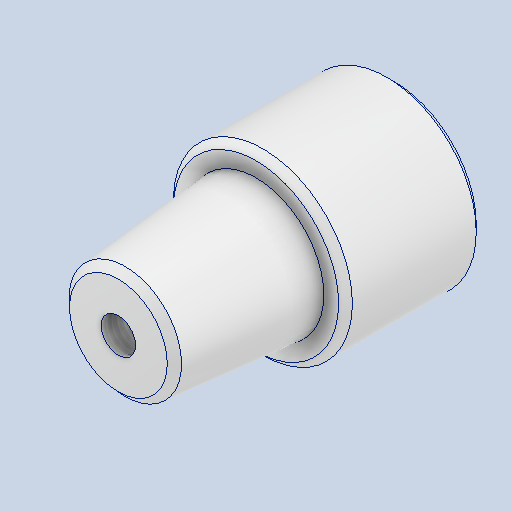
# Autodesk Inventor part: Linear Actuator Base Holder
Saved by Autodesk Inventor 2025.3 (Build 293356000, 356)
## iProperties
Created: 2025-10-10
Part Number: Linear Actuator Base Holder
Material: Aluminum 6061
Document SubType Name: Modeling
Designer: Haggag
Density: 2.7 g/cm^3
Appearance: Aluminum - Flat
Author: Haggag
Autodesk Inventor part; units mm, degrees
ref_plane "YZ Plane" through (0, 0, 0) normal (1, 0, 0) x (0, 1, 0)
ref_plane "XZ Plane" through (0, 0, 0) normal (0, 1, 0) x (-1, 0, 0)
ref_plane "XY Plane" through (0, 0, 0) normal (0, 0, 1) x (1, 0, 0)
sketch "Sketch1" plane through (0, 0, 0) normal (0, 0, 1) x (1, 0, 0)
  circle A0 centre (0, 0) radius 9.85
  circle A1 centre (0, 0) radius 13
  dimension "d0" = 19.7
  dimension "d1" = 26
  constraints: 2 centre point, 2 coincident
  measures "d0" diameter of A0
  measures "d1" diameter of A1
extrude "Extrusion1" add sketch "Sketch1" along normal blind 20
sketch "Sketch3" plane through (0, 0, 20) normal (0, 0, 1) x (1, 0, 0)
  circle A0 centre (0, 0) radius 9.85
  dimension "d21" = 19.7
  constraints: 1 centre point, 1 coincident
  measures "d21" diameter of A0
extrude "Extrusion3" add sketch "Sketch3" along normal blind 20 draft -5
chamfer "Chamfer1" distance 1 angle 45 1 edges at (-8.1002, 0, 40)
chamfer "Chamfer2" distance 1 angle 45 2 edges at (-13, 0, 20) (-13, 0, 0)
sketch "Sketch4" plane through (0, 0, 40) normal (0, 0, 1) x (1, 0, 0)
  circle A0 centre (0, 0) radius 2.5
  dimension "d16" = 5
  constraints: 1 centre point, 1 coincident
  measures "d16" diameter of A0
extrude "Extrusion4" cut sketch "Sketch4" against normal blind 19
thread "Thread1" size "M5x0.8" class "6H" standard "ANSI Metric M Profile" full length
body "Solid1"
